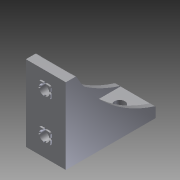
# Autodesk Inventor part: HBLFSSW5-SEThblfsn5
Saved by Autodesk Inventor 2011 SP1 (Build 150282100, 282)
## iProperties
Created: 2013-06-20
Part Number: HBLFSSW5-SEThblfsn5
Catalog Web Link: www.cadenas.de
Description: HBLFSN5, HBLFSNB5, HBLFSNM5, HBLFSNK5, HBLFSSW5, HBLFSSWB5, HBLFSDW5-Thin Reversal Brackets for Slot Width 6 Frames - For 20, 40mm Sections
Vendor: MISUMI
Document SubType Name: Modeling
Designer: PARTuser1
Manufacturer: MISUMI
Density: 1 g/cm^3
Category: PARTsolutions
Company: MISUMI
Title: HBLFSSW5-SEThblfsn5
Author: Cadenas PARTsolutions
Comments: Thin Reversal Brackets for Slot Width 6 Frames - For 20, 40mm Sections
PSOL_IDENT_0: {\\10.0.0.242\data_v8\23d-libs\misumi\metric\38_al_extrusions_blackets\5\hblfsn5.prj},251 {VTYP=3D},
PSOL_IDENT_1: {NB=HBLFSSW5-SEThblfsn5},{LINA=HBLFSSW5-SEThblfsn5},{NN=HBLFSN5, HBLFSNB5, HBLFSNM5, HBLFSNK5, HBLFS
PSOL_IDENT_2: SW5, HBLFSSWB5, HBLFSDW5},{DATE=28.02.2012 00:46:20},{GEOMDATE=28.01.2010 06:29:00},{VERSION=},{LINE
PSOL_IDENT_3: ID=50},{LINESUBID=-1},{WBVAR=ALT1,ALT2}  {NB=HBLFSSW5-SEThblfsn5},{LINA=HBLFSSW5-SEThblfsn5},{KT=2},
PSOL_IDENT_4: {PN=HBLFSSW5-SET},{TP=HBLFSSW5},{NOH=1},{NOHV=2},{MAT=JIS-ADC12},{ST=-},{TYPE=HBLFSSW5},{FEAT=Thin R
PSOL_IDENT_5: eversal Bracket},{ALT1=},{ALT2=-SET},{MASS=24},{AB=CBM5-10},{NOB=4},{AN=HNTT5-5},{NON=4},{AL=1470},{
PSOL_IDENT_6: W=20},{H=45},{DP=38},{T=5.0},{HDIS=15},{DPOS=12},{HH1=30},{BOLTX=0.0},{HV1=37},{BOLTY=0.0},{DIA=5.2}
PSOL_IDENT_7: ,{ALT1OPT='','w/o C (Mounting Holes for Cover)','-C','with C (Mounting Holes for Cover)'},{ALT2OPT=
PSOL_IDENT_8: '' , 'w/o Set Applicable Bolt & Nut' , '-SET' , 'with SET (Set Applicable Bolt & Nut)' , '-SST' , 'w
PSOL_IDENT_9: ith SST (Stainless Steel Set Applicable Bolt & Nut)' , '-SEP' , 'with SEP (Post Assembly Spring Nuts
PSOL_IDENT_10: Set Applicable Bolt & Nut)' , '-SSP' , 'with SSP (Post Assembly Spring Nuts, Stainless Steel Set Ap
PSOL_IDENT_11: plicable Bolt & Nut)' },{R=1},{R1=0.3},{APOSV=0},{VER=1},{PR=2},{TT=0.8},{T1=3}
SUPPLIER: MISUMI
ARTICLENO: HBLFSSW5-SEThblfsn5
BOMINFO: HBLFSSW5-SEThblfsn5
CREATOR: CADENAS GmbH
Autodesk Inventor part; units mm, degrees
ref_plane "YZ Plane" through (0, 0, 0) normal (1, 0, 0) x (0, 1, 0)
ref_plane "XZ Plane" through (0, 0, 0) normal (0, 1, 0) x (-1, 0, 0)
ref_plane "XY Plane" through (0, 0, 0) normal (0, 0, 1) x (1, 0, 0)
sketch "Sketch_15" plane through (0, 0, 0) normal (1, 0, 0) x (0, 1, 0)
  line L0 (0, 38) -> (0, 0)
  line L1 (0, 0) -> (45, 0)
  line L2 (45, 0) -> (45, 4.5286)
  arc A0 (45, 4.5286) -> (44.6364, 5.3) centre (44, 4.5286) ccw
  line L3 (44.6364, 5.3) -> (5.2771, 37.7714)
  arc A1 (5.2771, 37.7714) -> (4.6407, 38) centre (4.6407, 37) ccw
  line L4 (4.6407, 38) -> (0, 38)
  constraints: 10 end point, 4 point on circle, 2 centre point
extrude "Extrusion1" add sketch "Sketch_15" along normal mid plane 20
sketch "Sketch_16" plane through (0, 0, 0) normal (1, 0, 0) x (0, 1, 0)
  line L0 (5, 43) -> (5, 5)
  line L1 (5, 5) -> (50, 5)
  line L2 (50, 5) -> (50, 43)
  line L3 (50, 43) -> (5, 43)
  constraints: 8 end point
extrude "Extrusion2" cut sketch "Sketch_16" along normal mid plane 15
sketch "Sketch_28" plane through (0, 0, 0) normal (1, 0, 0) x (0, 1, 0)
  arc A0 (5.2771, 37.7714) -> (44.6364, 5.3) centre (64.787, 69.8148) ccw
  line L0 (44.6364, 5.3) -> (5.2771, 37.7714)
  constraints: 2 end point, 2 point on circle, 1 centre point
extrude "Extrusion3" cut sketch "Sketch_28" along normal mid plane 20
sketch "Sketch_6" plane through (0, 0, 0) normal (0, 1, 0) x (1, 0, 0)
  circle A0 centre (0, -10) radius 2.6
  constraints: 1 centre point
extrude "Extrusion4" cut sketch "Sketch_6" along normal blind 5
pattern_linear "Rectangular Pattern1" count 2 spacing 20 along (0, 0, 1) of "Extrusion4"
sketch "Sketch_8" plane through (0, 0, 0) normal (0, 0, 1) x (1, 0, 0)
  circle A0 centre (0, 22) radius 2.6
  constraints: 1 centre point
extrude "Extrusion5" cut sketch "Sketch_8" along normal blind 5
pattern_linear "Rectangular Pattern2" count 2 spacing 15 along (0, 1, 0) of "Extrusion5"
sketch "Sketch_1" plane through (0, 0, 0) normal (0, 1, 0) x (-1, 0, 0)
  line L0 (10, 0) -> (10, 38)
  line L1 (10, 38) -> (-10, 38)
  line L2 (-10, 38) -> (-10, 0)
  line L3 (-10, 0) -> (10, 0)
  constraints: 8 end point
extrude "Extrusion6" add sketch "Sketch_1" against normal blind 0.8
sketch "Sketch_10" plane through (0, 0, 0) normal (0, 0, 1) x (1, 0, 0)
  line L0 (-10, 0) -> (10, 0)
  line L1 (10, 0) -> (10, 45)
  line L2 (10, 45) -> (-10, 45)
  line L3 (-10, 45) -> (-10, 0)
  constraints: 8 end point
extrude "Extrusion7" add sketch "Sketch_10" against normal blind 0.8
sketch "Sketch_13" plane through (0, 0, 0) normal (0, 1, 0) x (-1, 0, 0)
  line L0 (10, 0) -> (10, 38)
  line L1 (10, 38) -> (-10, 38)
  line L2 (-10, 38) -> (-10, 0)
  line L3 (-10, 0) -> (10, 0)
  line L4 (-0.5, 33) -> (-2, 33)
  arc A0 (-2, 33) -> (-3, 32) centre (-2, 32) ccw
  line L5 (-3, 32) -> (-3, 30.5)
  line L6 (-3, 30.5) -> (-2.5515, 30.5)
  arc A1 (-0.5, 32.5515) -> (-2.5515, 30.5) centre (0, 30) ccw
  line L7 (-0.5, 32.5515) -> (-0.5, 33)
  line L8 (-0.5, 27) -> (-0.5, 27.4485)
  arc A2 (-2.5515, 29.5) -> (-0.5, 27.4485) centre (0, 30) ccw
  line L9 (-2.5515, 29.5) -> (-3, 29.5)
  line L10 (-3, 29.5) -> (-3, 28)
  arc A3 (-3, 28) -> (-2, 27) centre (-2, 28) ccw
  line L11 (-2, 27) -> (-0.5, 27)
  line L12 (-0.5, 13) -> (-2, 13)
  arc A4 (-2, 13) -> (-3, 12) centre (-2, 12) ccw
  line L13 (-3, 12) -> (-3, 10.5)
  line L14 (-3, 10.5) -> (-2.5515, 10.5)
  arc A5 (-0.5, 12.5515) -> (-2.5515, 10.5) centre (0, 10) ccw
  line L15 (-0.5, 12.5515) -> (-0.5, 13)
  line L16 (-0.5, 7) -> (-0.5, 7.4485)
  arc A6 (-2.5515, 9.5) -> (-0.5, 7.4485) centre (0, 10) ccw
  line L17 (-2.5515, 9.5) -> (-3, 9.5)
  line L18 (-3, 9.5) -> (-3, 8)
  arc A7 (-3, 8) -> (-2, 7) centre (-2, 8) ccw
  line L19 (-2, 7) -> (-0.5, 7)
  arc A8 (3, 32) -> (2, 33) centre (2, 32) ccw
  line L20 (2, 33) -> (0.5, 33)
  line L21 (0.5, 33) -> (0.5, 32.5515)
  arc A9 (2.5515, 30.5) -> (0.5, 32.5515) centre (0, 30) ccw
  line L22 (2.5515, 30.5) -> (3, 30.5)
  line L23 (3, 30.5) -> (3, 32)
  line L24 (3, 29.5) -> (2.5515, 29.5)
  arc A10 (0.5, 27.4485) -> (2.5515, 29.5) centre (0, 30) ccw
  line L25 (0.5, 27.4485) -> (0.5, 27)
  line L26 (0.5, 27) -> (2, 27)
  arc A11 (2, 27) -> (3, 28) centre (2, 28) ccw
  line L27 (3, 28) -> (3, 29.5)
  arc A12 (3, 12) -> (2, 13) centre (2, 12) ccw
  line L28 (2, 13) -> (0.5, 13)
  line L29 (0.5, 13) -> (0.5, 12.5515)
  arc A13 (2.5515, 10.5) -> (0.5, 12.5515) centre (0, 10) ccw
  line L30 (2.5515, 10.5) -> (3, 10.5)
  line L31 (3, 10.5) -> (3, 12)
  line L32 (3, 9.5) -> (2.5515, 9.5)
  arc A14 (0.5, 7.4485) -> (2.5515, 9.5) centre (0, 10) ccw
  line L33 (0.5, 7.4485) -> (0.5, 7)
  line L34 (0.5, 7) -> (2, 7)
  arc A15 (2, 7) -> (3, 8) centre (2, 8) ccw
  line L35 (3, 8) -> (3, 9.5)
  constraints: 72 end point, 32 point on circle, 16 centre point
extrude "Extrusion8" cut sketch "Sketch_13" against normal blind 0.8
sketch "Sketch_26" plane through (0, 0, 0) normal (0, 0, 1) x (1, 0, 0)
  line L0 (-10, 45) -> (-10, 0)
  line L1 (-10, 0) -> (10, 0)
  line L2 (10, 0) -> (10, 45)
  line L3 (10, 45) -> (-10, 45)
  arc A0 (-3, 27.3) -> (-2.7, 27) centre (-2.7, 27.3) ccw
  line L4 (-2.7, 27) -> (2.7, 27)
  arc A1 (2.7, 27) -> (3, 27.3) centre (2.7, 27.3) ccw
  line L5 (3, 27.3) -> (3, 32.7)
  arc A2 (3, 32.7) -> (2.7, 33) centre (2.7, 32.7) ccw
  line L6 (2.7, 33) -> (-2.7, 33)
  arc A3 (-2.7, 33) -> (-3, 32.7) centre (-2.7, 32.7) ccw
  line L7 (-3, 32.7) -> (-3, 27.3)
  arc A4 (-3, 3.3) -> (-2.7, 3) centre (-2.7, 3.3) ccw
  line L8 (-2.7, 3) -> (2.7, 3)
  arc A5 (2.7, 3) -> (3, 3.3) centre (2.7, 3.3) ccw
  line L9 (3, 3.3) -> (3, 7.7)
  arc A6 (3, 7.7) -> (2.7, 8) centre (2.7, 7.7) ccw
  line L10 (2.7, 8) -> (-2.7, 8)
  arc A7 (-2.7, 8) -> (-3, 7.7) centre (-2.7, 7.7) ccw
  line L11 (-3, 7.7) -> (-3, 3.3)
  constraints: 24 end point, 16 point on circle, 8 centre point
extrude "Extrusion9" cut sketch "Sketch_26" against normal blind 1.25
ref_plane "to_bolt_row_8_to_9_1_XY" through (0, 22, 5) normal (0, 0, 1) x (1, 0, 0)
ref_plane "to_bolt_row_8_to_9_1_YZ" through (0, 22, 5) normal (1, 0, 0) x (0, 1, 0)
ref_plane "to_bolt_row_8_to_9_1_ZX" through (0, 22, 5) normal (0, 1, 0) x (0, 0, 1)
ref_plane "to_bolt_row_8_to_9_2_XY" through (0, 37, 5) normal (0, 0, 1) x (1, 0, 0)
ref_plane "to_bolt_row_8_to_9_2_YZ" through (0, 37, 5) normal (1, 0, 0) x (0, 1, 0)
ref_plane "to_bolt_row_8_to_9_2_ZX" through (0, 37, 5) normal (0, 1, 0) x (0, 0, 1)
ref_plane "to_bolt_row_8_9_base_2_XY" through (0, 5, 30) normal (0, 1, 0) x (1, 0, 0)
ref_plane "to_bolt_row_8_9_base_2_YZ" through (0, 5, 30) normal (1, 0, 0) x (0, 0, -1)
ref_plane "to_bolt_row_8_9_base_2_ZX" through (0, 5, 30) normal (0, 0, -1) x (0, 1, 0)
ref_plane "to_bolt_row_8_9_base_1_XY" through (0, 5, 10) normal (0, 1, 0) x (1, 0, 0)
ref_plane "to_bolt_row_8_9_base_1_YZ" through (0, 5, 10) normal (1, 0, 0) x (0, 0, -1)
ref_plane "to_bolt_row_8_9_base_1_ZX" through (0, 5, 10) normal (0, 0, -1) x (0, 1, 0)
ref_plane "to_nut_row_8_to_9_2_XY" through (0, 37, -2) normal (0, 0, 1) x (1, 0, 0)
ref_plane "to_nut_row_8_to_9_2_YZ" through (0, 37, -2) normal (1, 0, 0) x (0, 1, 0)
ref_plane "to_nut_row_8_to_9_2_ZX" through (0, 37, -2) normal (0, 1, 0) x (0, 0, 1)
ref_plane "to_nut_row_8_to_9_1_XY" through (0, 22, -2) normal (0, 0, 1) x (1, 0, 0)
ref_plane "to_nut_row_8_to_9_1_YZ" through (0, 22, -2) normal (1, 0, 0) x (0, 1, 0)
ref_plane "to_nut_row_8_to_9_1_ZX" through (0, 22, -2) normal (0, 1, 0) x (0, 0, 1)
ref_plane "to_nut_row_8_9_base_2_XY" through (0, -2, 30) normal (0, 1, 0) x (1, 0, 0)
ref_plane "to_nut_row_8_9_base_2_YZ" through (0, -2, 30) normal (1, 0, 0) x (0, 0, -1)
ref_plane "to_nut_row_8_9_base_2_ZX" through (0, -2, 30) normal (0, 0, -1) x (0, 1, 0)
ref_plane "to_nut_row_8_9_base_1_XY" through (0, -2, 10) normal (0, 1, 0) x (1, 0, 0)
ref_plane "to_nut_row_8_9_base_1_YZ" through (0, -2, 10) normal (1, 0, 0) x (0, 0, -1)
ref_plane "to_nut_row_8_9_base_1_ZX" through (0, -2, 10) normal (0, 0, -1) x (0, 1, 0)
ref_plane "bracket_to_dummy_XY" through (0, 0, 0) normal (0, 1, 0) x (1, 0, 0)
ref_plane "bracket_to_dummy_YZ" through (0, 0, 0) normal (1, 0, 0) x (0, 0, -1)
ref_plane "bracket_to_dummy_ZX" through (0, 0, 0) normal (0, 0, -1) x (0, 1, 0)
ref_plane "bracket_to_bolt_XY" through (1, 37, 0) normal (0, 0, 1) x (1, 0, 0)
ref_plane "bracket_to_bolt_YZ" through (1, 37, 0) normal (1, 0, 0) x (0, 1, 0)
ref_plane "bracket_to_bolt_ZX" through (1, 37, 0) normal (0, 1, 0) x (0, 0, 1)
body "Solid1"
